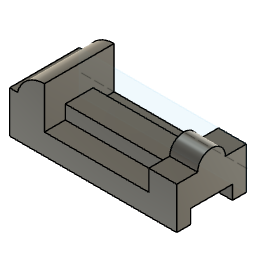
design 2 v1 (Autodesk Fusion 360 design; units mm, degrees)
Autodesk Fusion 360 part; units mm, degrees
note: some values were not read from the file. Set by a fixed rule: which sketch regions a step uses.
sketch "Sketch1" plane through (0, 0, 0) normal (0, 0, 1) x (1, 0, 0) in component "block"
  line L0 (60, -25) -> (-60, -25)
  line L1 (-60, -25) -> (-60, 25)
  line L2 (-60, 25) -> (60, 25)
  line L3 (60, 25) -> (60, -25)
  line L4 (60, -25) -> (-60, 25) construction
  line L5 (-60, -25) -> (60, 25) construction
  dimension "d1" = 120
  dimension "d2" = 50
  constraint horizontal L0
  constraint perpendicular L0 L1
  constraint parallel L0 L2
  constraint parallel L1 L3
  constraint coincident L4 origin
  constraint coincident L5 origin
  measures "d1" distance of L1.end L2.end
  measures "d2" distance of L0.end L1.end
extrude "Extrude1" add sketch "Sketch1" against normal blind 10 makes body 1 in component "block"
move_face "OffsetFaces1" offset 20 1 faces at (20, -8.3333, 0) on bodies 1 in component "block"
sketch "Sketch2" plane through (60, 0, 0) normal (1, 0, 0) x (0, 1, 0) in component "block"
  line L0 (25, 20) -> (-25, 20)
  line L1 (-25, 20) -> (-25, -10)
  line L2 (-25, -10) -> (25, -10)
  line L3 (25, -10) -> (25, 20)
  line L4 (-15, 0) -> (-15, -10)
  line L5 (15, 0) -> (15, -10)
  line L6 (-15, 0) -> (15, 0)
  line L7 (15, -10) -> (-15, -10)
  constraint coincident L2 L4.end
  constraint perpendicular L2 L4
  constraint coincident L2 L5.end
  constraint perpendicular L2 L5
  constraint perpendicular L5 L6
extrude "Extrude2" cut sketch "Sketch2" against normal blind 120 contours L2 L4 L5 L6 L7 bodies 1 in component "block"
sketch "Sketch3" plane through (0, 25, 0) normal (0, 1, 0) x (-1, 0, 0) in component "block"
  line L0 (60, 20) -> (-60, 20)
  line L1 (-60, 20) -> (-60, -10)
  line L2 (-60, -10) -> (60, -10)
  line L3 (60, -10) -> (60, 20)
  line L4 (-60, 5) -> (60, 5) construction
  constraint midpoint L1 L4.start
  constraint midpoint L3 L4.end
sketch "Sketch4" plane through (0, 0, 20) normal (0, 0, 1) x (-1, 0, 0) in component "block"
  line L0 (-60, -25) -> (60, -25)
  line L1 (60, -25) -> (60, 25)
  line L2 (60, 25) -> (-60, 25)
  line L3 (-60, 25) -> (-60, -25)
  line L4 (35, -25) -> (35, 25)
  line L5 (-40, -25) -> (-40, 25)
  constraint coincident L0 L4.start
  constraint coincident L2 L4.end
  constraint perpendicular L2 L4
  constraint coincident L0 L5.start
  constraint coincident L2 L5.end
  constraint perpendicular L2 L5
sketch "Sketch5" plane through (-60, 0, 0) normal (-1, 0, 0) x (0, -1, 0) in component "block"
  line L0 (15, 0) -> (15, -10)
  line L1 (15, -10) -> (25, -10)
  line L2 (25, -10) -> (25, 20)
  line L3 (25, 20) -> (-25, 20)
  line L4 (-25, 20) -> (-25, -10)
  line L5 (-25, -10) -> (-15, -10)
  line L6 (-15, -10) -> (-15, 0)
  line L7 (-15, 0) -> (15, 0)
  line L8 (-10, 0) -> (-10, 15)
  line L9 (-10, 15) -> (10, 15)
  line L10 (10, 15) -> (10, 0)
  constraint coincident L7 L8.start
  constraint perpendicular L7 L8
  constraint perpendicular L8 L9
  constraint coincident L7 L10.end
  constraint perpendicular L7 L10
extrude "Extrude3" cut sketch "Sketch5" against normal blind 25 contours L7 L8 L9 L10 bodies 1 in component "block"
sketch "Sketch6" plane through (0, -25, 0) normal (0, -1, 0) x (1, 0, 0) in component "block"
  line L0 (60, 20) -> (-60, 20)
  line L1 (-60, 20) -> (-60, -10)
  line L2 (-60, -10) -> (60, -10)
  line L3 (60, -10) -> (60, 20)
  line L4 (-60, 5) -> (-35, 5)
  line L5 (-35, 5) -> (-35, 20)
  circle A0 centre (-35, 15) radius 20
  line L6 (-35, 20) -> (-35, 35)
  constraint horizontal L4
  constraint coincident L0 L5.end
  constraint perpendicular L0 L5
  constraint coincident L5 A0.centre
  constraint coincident A0 L6.end
  constraint perpendicular L0 L6
extrude "Extrude4" cut sketch "Sketch4" against normal blind 15 contours L0 L2 L4 L5 bodies 1 in component "block"
sketch "Sketch7" plane through (0, 0, 5) normal (0, 0, 1) x (-1, 0, 0) in component "block"
  line L0 (35, 10) -> (35, 25)
  line L1 (35, 25) -> (-40, 25)
  line L2 (-40, 25) -> (-40, -25)
  line L3 (-40, -25) -> (35, -25)
  line L4 (35, -25) -> (35, -10)
  line L5 (35, -10) -> (35, 10)
  line L6 (35, -10) -> (-40, -10)
  line L7 (35, 10) -> (-40, 10)
  constraint coincident L4.end L5.start
  constraint coincident L2 L6.end
  constraint perpendicular L2 L6
  constraint coincident L0.start L5.end
  constraint coincident L2 L7.end
  constraint perpendicular L2 L7
extrude "Extrude5" add sketch "Sketch7" along normal blind 10 separate body contours L2 L5 L6 L7 makes body 2 in component "block"
extrude "Extrude6" add sketch "Sketch6" against normal blind 50 contours L0 A0 L6 picked at (-35.9729, 29.9286) bodies 1 in component "block"
sketch "Sketch8" plane through (60, 0, 0) normal (1, 0, 0) x (0, 1, 0) in component "block"
  line L0 (-15, -10) -> (-15, 0)
  line L1 (-15, 0) -> (15, 0)
  line L2 (15, 0) -> (15, -10)
  line L3 (15, -10) -> (25, -10)
  line L4 (25, -10) -> (25, 20)
  line L5 (25, 20) -> (-25, 20)
  line L6 (-25, 20) -> (-25, -10)
  line L7 (-25, -10) -> (-15, -10)
  circle A0 centre (0, 20) radius 10
  constraint midpoint L5 A0.centre
extrude "Extrude7" add sketch "Sketch8" against normal blind 20 contours L5 A0 picked at (2.0783, 22.6061) bodies 1 in component "block"
component "block" placed x (1, 0, 0) y (0, 1, 0) z (0, 0, 1) at (0, 0, 0)
